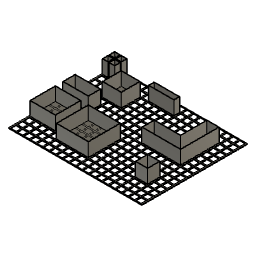
Grid (Autodesk Fusion 360 design; units mm, degrees)
Autodesk Fusion 360 part; units mm, degrees
note: some values were not read from the file. Set by a fixed rule: which face or edge a step refers to.
(part 1 of 2)
sketch "Sketch4" plane through (0, 0, 0) normal (0, 0, 1) x (1, 0, 0)
  line L0 (0, 0) -> (486, 0)
  line L1 (486, 0) -> (486, 385)
  line L2 (486, 385) -> (0, 385)
  line L3 (0, 385) -> (0, 0)
  line L4 (5, 2.5) -> (0, 2.5) construction
  line L5 (5, 2.5) -> (5, 0) construction
  line L6 (5, 2.5) -> (25, 2.5)
  line L7 (25, 2.5) -> (25, 22.5)
  line L8 (25, 22.5) -> (5, 22.5)
  line L9 (5, 22.5) -> (5, 2.5)
  line L10 (49, 22.5) -> (29, 22.5)
  line L11 (29, 22.5) -> (29, 2.5)
  line L12 (29, 2.5) -> (49, 2.5)
  line L13 (49, 2.5) -> (49, 22.5)
  line L14 (73, 22.5) -> (53, 22.5)
  line L15 (53, 22.5) -> (53, 2.5)
  line L16 (53, 2.5) -> (73, 2.5)
  line L17 (73, 2.5) -> (73, 22.5)
  line L18 (97, 22.5) -> (77, 22.5)
  line L19 (77, 22.5) -> (77, 2.5)
  line L20 (77, 2.5) -> (97, 2.5)
  line L21 (97, 2.5) -> (97, 22.5)
  line L22 (25, 46.5) -> (5, 46.5)
  line L23 (5, 46.5) -> (5, 26.5)
  line L24 (5, 26.5) -> (25, 26.5)
  line L25 (25, 26.5) -> (25, 46.5)
  line L26 (49, 46.5) -> (29, 46.5)
  line L27 (29, 46.5) -> (29, 26.5)
  line L28 (29, 26.5) -> (49, 26.5)
  line L29 (49, 26.5) -> (49, 46.5)
  line L30 (73, 46.5) -> (53, 46.5)
  line L31 (53, 46.5) -> (53, 26.5)
  line L32 (53, 26.5) -> (73, 26.5)
  line L33 (73, 26.5) -> (73, 46.5)
  line L34 (97, 46.5) -> (77, 46.5)
  line L35 (77, 46.5) -> (77, 26.5)
  line L36 (77, 26.5) -> (97, 26.5)
  line L37 (97, 26.5) -> (97, 46.5)
  line L38 (25, 70.5) -> (5, 70.5)
  line L39 (5, 70.5) -> (5, 50.5)
  line L40 (5, 50.5) -> (25, 50.5)
  line L41 (25, 50.5) -> (25, 70.5)
  line L42 (49, 70.5) -> (29, 70.5)
  line L43 (29, 70.5) -> (29, 50.5)
  line L44 (29, 50.5) -> (49, 50.5)
  line L45 (49, 50.5) -> (49, 70.5)
  line L46 (73, 70.5) -> (53, 70.5)
  line L47 (53, 70.5) -> (53, 50.5)
  line L48 (53, 50.5) -> (73, 50.5)
  line L49 (73, 50.5) -> (73, 70.5)
  line L50 (97, 70.5) -> (77, 70.5)
  line L51 (77, 70.5) -> (77, 50.5)
  line L52 (77, 50.5) -> (97, 50.5)
  line L53 (97, 50.5) -> (97, 70.5)
  line L54 (25, 94.5) -> (5, 94.5)
  line L55 (5, 94.5) -> (5, 74.5)
  line L56 (5, 74.5) -> (25, 74.5)
  line L57 (25, 74.5) -> (25, 94.5)
  line L58 (49, 94.5) -> (29, 94.5)
  line L59 (29, 94.5) -> (29, 74.5)
  line L60 (29, 74.5) -> (49, 74.5)
  line L61 (49, 74.5) -> (49, 94.5)
  line L62 (73, 94.5) -> (53, 94.5)
  line L63 (53, 94.5) -> (53, 74.5)
  line L64 (53, 74.5) -> (73, 74.5)
  line L65 (73, 74.5) -> (73, 94.5)
  line L66 (97, 94.5) -> (77, 94.5)
  line L67 (77, 94.5) -> (77, 74.5)
  line L68 (77, 74.5) -> (97, 74.5)
  line L69 (97, 74.5) -> (97, 94.5)
  line L70 (121, 22.5) -> (101, 22.5)
  line L71 (101, 22.5) -> (101, 2.5)
  line L72 (101, 2.5) -> (121, 2.5)
  line L73 (121, 2.5) -> (121, 22.5)
  line L74 (145, 22.5) -> (125, 22.5)
  line L75 (125, 22.5) -> (125, 2.5)
  line L76 (125, 2.5) -> (145, 2.5)
  line L77 (145, 2.5) -> (145, 22.5)
  line L78 (169, 22.5) -> (149, 22.5)
  line L79 (149, 22.5) -> (149, 2.5)
  line L80 (149, 2.5) -> (169, 2.5)
  line L81 (169, 2.5) -> (169, 22.5)
  line L82 (193, 22.5) -> (173, 22.5)
  line L83 (173, 22.5) -> (173, 2.5)
  line L84 (173, 2.5) -> (193, 2.5)
  line L85 (193, 2.5) -> (193, 22.5)
  line L86 (217, 22.5) -> (197, 22.5)
  line L87 (197, 22.5) -> (197, 2.5)
  line L88 (197, 2.5) -> (217, 2.5)
  line L89 (217, 2.5) -> (217, 22.5)
  line L90 (241, 22.5) -> (221, 22.5)
  line L91 (221, 22.5) -> (221, 2.5)
  line L92 (221, 2.5) -> (241, 2.5)
  line L93 (241, 2.5) -> (241, 22.5)
  line L94 (265, 22.5) -> (245, 22.5)
  line L95 (245, 22.5) -> (245, 2.5)
  line L96 (245, 2.5) -> (265, 2.5)
  line L97 (265, 2.5) -> (265, 22.5)
  line L98 (289, 22.5) -> (269, 22.5)
  line L99 (269, 22.5) -> (269, 2.5)
  line L100 (269, 2.5) -> (289, 2.5)
  line L101 (289, 2.5) -> (289, 22.5)
  line L102 (121, 46.5) -> (101, 46.5)
  line L103 (101, 46.5) -> (101, 26.5)
  line L104 (101, 26.5) -> (121, 26.5)
  line L105 (121, 26.5) -> (121, 46.5)
  line L106 (145, 46.5) -> (125, 46.5)
  line L107 (125, 46.5) -> (125, 26.5)
  line L108 (125, 26.5) -> (145, 26.5)
  line L109 (145, 26.5) -> (145, 46.5)
  line L110 (169, 46.5) -> (149, 46.5)
  line L111 (149, 46.5) -> (149, 26.5)
  line L112 (149, 26.5) -> (169, 26.5)
  line L113 (169, 26.5) -> (169, 46.5)
  line L114 (193, 46.5) -> (173, 46.5)
  line L115 (173, 46.5) -> (173, 26.5)
  line L116 (173, 26.5) -> (193, 26.5)
  line L117 (193, 26.5) -> (193, 46.5)
  line L118 (217, 46.5) -> (197, 46.5)
  line L119 (197, 46.5) -> (197, 26.5)
  line L120 (197, 26.5) -> (217, 26.5)
  line L121 (217, 26.5) -> (217, 46.5)
  line L122 (241, 46.5) -> (221, 46.5)
  line L123 (221, 46.5) -> (221, 26.5)
  line L124 (221, 26.5) -> (241, 26.5)
  line L125 (241, 26.5) -> (241, 46.5)
  line L126 (265, 46.5) -> (245, 46.5)
  line L127 (245, 46.5) -> (245, 26.5)
  line L128 (245, 26.5) -> (265, 26.5)
  line L129 (265, 26.5) -> (265, 46.5)
  line L130 (289, 46.5) -> (269, 46.5)
  line L131 (269, 46.5) -> (269, 26.5)
  line L132 (269, 26.5) -> (289, 26.5)
  line L133 (289, 26.5) -> (289, 46.5)
  line L134 (121, 70.5) -> (101, 70.5)
  line L135 (101, 70.5) -> (101, 50.5)
  line L136 (101, 50.5) -> (121, 50.5)
  line L137 (121, 50.5) -> (121, 70.5)
  line L138 (145, 70.5) -> (125, 70.5)
  line L139 (125, 70.5) -> (125, 50.5)
  line L140 (125, 50.5) -> (145, 50.5)
  line L141 (145, 50.5) -> (145, 70.5)
  line L142 (169, 70.5) -> (149, 70.5)
  line L143 (149, 70.5) -> (149, 50.5)
  line L144 (149, 50.5) -> (169, 50.5)
  line L145 (169, 50.5) -> (169, 70.5)
  line L146 (193, 70.5) -> (173, 70.5)
  line L147 (173, 70.5) -> (173, 50.5)
  line L148 (173, 50.5) -> (193, 50.5)
  line L149 (193, 50.5) -> (193, 70.5)
  line L150 (217, 70.5) -> (197, 70.5)
  line L151 (197, 70.5) -> (197, 50.5)
  line L152 (197, 50.5) -> (217, 50.5)
  line L153 (217, 50.5) -> (217, 70.5)
  line L154 (241, 70.5) -> (221, 70.5)
  line L155 (221, 70.5) -> (221, 50.5)
  line L156 (221, 50.5) -> (241, 50.5)
  line L157 (241, 50.5) -> (241, 70.5)
  line L158 (265, 70.5) -> (245, 70.5)
  line L159 (245, 70.5) -> (245, 50.5)
  line L160 (245, 50.5) -> (265, 50.5)
  line L161 (265, 50.5) -> (265, 70.5)
  line L162 (289, 70.5) -> (269, 70.5)
  line L163 (269, 70.5) -> (269, 50.5)
  line L164 (269, 50.5) -> (289, 50.5)
  line L165 (289, 50.5) -> (289, 70.5)
  line L166 (121, 94.5) -> (101, 94.5)
  line L167 (101, 94.5) -> (101, 74.5)
  line L168 (101, 74.5) -> (121, 74.5)
  line L169 (121, 74.5) -> (121, 94.5)
  line L170 (145, 94.5) -> (125, 94.5)
  line L171 (125, 94.5) -> (125, 74.5)
  line L172 (125, 74.5) -> (145, 74.5)
  line L173 (145, 74.5) -> (145, 94.5)
  line L174 (169, 94.5) -> (149, 94.5)
  line L175 (149, 94.5) -> (149, 74.5)
  line L176 (149, 74.5) -> (169, 74.5)
  line L177 (169, 74.5) -> (169, 94.5)
  line L178 (193, 94.5) -> (173, 94.5)
  line L179 (173, 94.5) -> (173, 74.5)
  line L180 (173, 74.5) -> (193, 74.5)
  line L181 (193, 74.5) -> (193, 94.5)
  line L182 (217, 94.5) -> (197, 94.5)
  line L183 (197, 94.5) -> (197, 74.5)
  line L184 (197, 74.5) -> (217, 74.5)
  line L185 (217, 74.5) -> (217, 94.5)
  line L186 (241, 94.5) -> (221, 94.5)
  line L187 (221, 94.5) -> (221, 74.5)
  line L188 (221, 74.5) -> (241, 74.5)
  line L189 (241, 74.5) -> (241, 94.5)
  line L190 (265, 94.5) -> (245, 94.5)
  line L191 (245, 94.5) -> (245, 74.5)
  line L192 (245, 74.5) -> (265, 74.5)
  line L193 (265, 74.5) -> (265, 94.5)
  line L194 (289, 94.5) -> (269, 94.5)
  line L195 (269, 94.5) -> (269, 74.5)
  line L196 (269, 74.5) -> (289, 74.5)
  line L197 (289, 74.5) -> (289, 94.5)
  line L198 (25, 118.5) -> (5, 118.5)
  line L199 (5, 118.5) -> (5, 98.5)
  line L200 (5, 98.5) -> (25, 98.5)
  line L201 (25, 98.5) -> (25, 118.5)
  line L202 (49, 118.5) -> (29, 118.5)
  line L203 (29, 118.5) -> (29, 98.5)
  line L204 (29, 98.5) -> (49, 98.5)
  line L205 (49, 98.5) -> (49, 118.5)
  line L206 (73, 118.5) -> (53, 118.5)
  line L207 (53, 118.5) -> (53, 98.5)
  line L208 (53, 98.5) -> (73, 98.5)
  line L209 (73, 98.5) -> (73, 118.5)
  line L210 (97, 118.5) -> (77, 118.5)
  line L211 (77, 118.5) -> (77, 98.5)
  line L212 (77, 98.5) -> (97, 98.5)
  line L213 (97, 98.5) -> (97, 118.5)
  line L214 (121, 118.5) -> (101, 118.5)
  line L215 (101, 118.5) -> (101, 98.5)
  line L216 (101, 98.5) -> (121, 98.5)
  line L217 (121, 98.5) -> (121, 118.5)
  line L218 (145, 118.5) -> (125, 118.5)
  line L219 (125, 118.5) -> (125, 98.5)
  line L220 (125, 98.5) -> (145, 98.5)
  line L221 (145, 98.5) -> (145, 118.5)
  line L222 (169, 118.5) -> (149, 118.5)
  line L223 (149, 118.5) -> (149, 98.5)
  line L224 (149, 98.5) -> (169, 98.5)
  line L225 (169, 98.5) -> (169, 118.5)
  line L226 (193, 118.5) -> (173, 118.5)
  line L227 (173, 118.5) -> (173, 98.5)
  line L228 (173, 98.5) -> (193, 98.5)
  line L229 (193, 98.5) -> (193, 118.5)
  line L230 (217, 118.5) -> (197, 118.5)
  line L231 (197, 118.5) -> (197, 98.5)
  line L232 (197, 98.5) -> (217, 98.5)
  line L233 (217, 98.5) -> (217, 118.5)
  line L234 (241, 118.5) -> (221, 118.5)
  line L235 (221, 118.5) -> (221, 98.5)
  line L236 (221, 98.5) -> (241, 98.5)
  line L237 (241, 98.5) -> (241, 118.5)
  line L238 (265, 118.5) -> (245, 118.5)
  line L239 (245, 118.5) -> (245, 98.5)
  line L240 (245, 98.5) -> (265, 98.5)
  line L241 (265, 98.5) -> (265, 118.5)
  line L242 (289, 118.5) -> (269, 118.5)
  line L243 (269, 118.5) -> (269, 98.5)
  line L244 (269, 98.5) -> (289, 98.5)
  line L245 (289, 98.5) -> (289, 118.5)
  line L246 (25, 142.5) -> (5, 142.5)
  line L247 (5, 142.5) -> (5, 122.5)
  line L248 (5, 122.5) -> (25, 122.5)
  line L249 (25, 122.5) -> (25, 142.5)
  line L250 (49, 142.5) -> (29, 142.5)
  line L251 (29, 142.5) -> (29, 122.5)
  line L252 (29, 122.5) -> (49, 122.5)
  line L253 (49, 122.5) -> (49, 142.5)
  line L254 (73, 142.5) -> (53, 142.5)
  line L255 (53, 142.5) -> (53, 122.5)
  line L256 (53, 122.5) -> (73, 122.5)
  line L257 (73, 122.5) -> (73, 142.5)
  line L258 (97, 142.5) -> (77, 142.5)
  line L259 (77, 142.5) -> (77, 122.5)
  line L260 (77, 122.5) -> (97, 122.5)
  line L261 (97, 122.5) -> (97, 142.5)
  line L262 (121, 142.5) -> (101, 142.5)
  line L263 (101, 142.5) -> (101, 122.5)
  line L264 (101, 122.5) -> (121, 122.5)
  line L265 (121, 122.5) -> (121, 142.5)
  line L266 (145, 142.5) -> (125, 142.5)
  line L267 (125, 142.5) -> (125, 122.5)
  line L268 (125, 122.5) -> (145, 122.5)
  line L269 (145, 122.5) -> (145, 142.5)
  line L270 (169, 142.5) -> (149, 142.5)
  line L271 (149, 142.5) -> (149, 122.5)
  line L272 (149, 122.5) -> (169, 122.5)
  line L273 (169, 122.5) -> (169, 142.5)
  line L274 (193, 142.5) -> (173, 142.5)
  line L275 (173, 142.5) -> (173, 122.5)
  line L276 (173, 122.5) -> (193, 122.5)
  line L277 (193, 122.5) -> (193, 142.5)
  line L278 (217, 142.5) -> (197, 142.5)
  line L279 (197, 142.5) -> (197, 122.5)
  line L280 (197, 122.5) -> (217, 122.5)
  line L281 (217, 122.5) -> (217, 142.5)
  line L282 (241, 142.5) -> (221, 142.5)
  line L283 (221, 142.5) -> (221, 122.5)
  line L284 (221, 122.5) -> (241, 122.5)
  line L285 (241, 122.5) -> (241, 142.5)
  line L286 (265, 142.5) -> (245, 142.5)
  line L287 (245, 142.5) -> (245, 122.5)
  line L288 (245, 122.5) -> (265, 122.5)
  line L289 (265, 122.5) -> (265, 142.5)
  line L290 (289, 142.5) -> (269, 142.5)
  line L291 (269, 142.5) -> (269, 122.5)
  line L292 (269, 122.5) -> (289, 122.5)
  line L293 (289, 122.5) -> (289, 142.5)
  line L294 (25, 166.5) -> (5, 166.5)
  line L295 (5, 166.5) -> (5, 146.5)
  line L296 (5, 146.5) -> (25, 146.5)
  line L297 (25, 146.5) -> (25, 166.5)
  line L298 (49, 166.5) -> (29, 166.5)
  line L299 (29, 166.5) -> (29, 146.5)
  line L300 (29, 146.5) -> (49, 146.5)
  line L301 (49, 146.5) -> (49, 166.5)
  line L302 (73, 166.5) -> (53, 166.5)
  line L303 (53, 166.5) -> (53, 146.5)
  line L304 (53, 146.5) -> (73, 146.5)
  line L305 (73, 146.5) -> (73, 166.5)
  line L306 (97, 166.5) -> (77, 166.5)
  line L307 (77, 166.5) -> (77, 146.5)
  line L308 (77, 146.5) -> (97, 146.5)
  line L309 (97, 146.5) -> (97, 166.5)
  line L310 (121, 166.5) -> (101, 166.5)
  line L311 (101, 166.5) -> (101, 146.5)
  line L312 (101, 146.5) -> (121, 146.5)
  line L313 (121, 146.5) -> (121, 166.5)
  line L314 (145, 166.5) -> (125, 166.5)
  line L315 (125, 166.5) -> (125, 146.5)
  line L316 (125, 146.5) -> (145, 146.5)
  line L317 (145, 146.5) -> (145, 166.5)
  line L318 (169, 166.5) -> (149, 166.5)
  line L319 (149, 166.5) -> (149, 146.5)
  line L320 (149, 146.5) -> (169, 146.5)
  line L321 (169, 146.5) -> (169, 166.5)
  line L322 (193, 166.5) -> (173, 166.5)
  line L323 (173, 166.5) -> (173, 146.5)
  line L324 (173, 146.5) -> (193, 146.5)
  line L325 (193, 146.5) -> (193, 166.5)
  line L326 (217, 166.5) -> (197, 166.5)
  line L327 (197, 166.5) -> (197, 146.5)
  line L328 (197, 146.5) -> (217, 146.5)
  line L329 (217, 146.5) -> (217, 166.5)
  line L330 (241, 166.5) -> (221, 166.5)
  line L331 (221, 166.5) -> (221, 146.5)
  line L332 (221, 146.5) -> (241, 146.5)
  line L333 (241, 146.5) -> (241, 166.5)
  line L334 (265, 166.5) -> (245, 166.5)
  line L335 (245, 166.5) -> (245, 146.5)
  line L336 (245, 146.5) -> (265, 146.5)
  line L337 (265, 146.5) -> (265, 166.5)
  line L338 (289, 166.5) -> (269, 166.5)
  line L339 (269, 166.5) -> (269, 146.5)
  line L340 (269, 146.5) -> (289, 146.5)
  line L341 (289, 146.5) -> (289, 166.5)
  line L342 (25, 190.5) -> (5, 190.5)
  line L343 (5, 190.5) -> (5, 170.5)
  line L344 (5, 170.5) -> (25, 170.5)
  line L345 (25, 170.5) -> (25, 190.5)
  line L346 (49, 190.5) -> (29, 190.5)
  line L347 (29, 190.5) -> (29, 170.5)
  line L348 (29, 170.5) -> (49, 170.5)
  line L349 (49, 170.5) -> (49, 190.5)
  line L350 (73, 190.5) -> (53, 190.5)
  line L351 (53, 190.5) -> (53, 170.5)
  line L352 (53, 170.5) -> (73, 170.5)
  line L353 (73, 170.5) -> (73, 190.5)
  line L354 (97, 190.5) -> (77, 190.5)
  line L355 (77, 190.5) -> (77, 170.5)
  line L356 (77, 170.5) -> (97, 170.5)
  line L357 (97, 170.5) -> (97, 190.5)
  line L358 (121, 190.5) -> (101, 190.5)
  line L359 (101, 190.5) -> (101, 170.5)
  line L360 (101, 170.5) -> (121, 170.5)
  line L361 (121, 170.5) -> (121, 190.5)
  line L362 (145, 190.5) -> (125, 190.5)
  line L363 (125, 190.5) -> (125, 170.5)
  line L364 (125, 170.5) -> (145, 170.5)
  line L365 (145, 170.5) -> (145, 190.5)
  line L366 (169, 190.5) -> (149, 190.5)
  line L367 (149, 190.5) -> (149, 170.5)
  line L368 (149, 170.5) -> (169, 170.5)
  line L369 (169, 170.5) -> (169, 190.5)
  line L370 (193, 190.5) -> (173, 190.5)
  line L371 (173, 190.5) -> (173, 170.5)
  line L372 (173, 170.5) -> (193, 170.5)
  line L373 (193, 170.5) -> (193, 190.5)
  line L374 (217, 190.5) -> (197, 190.5)
  line L375 (197, 190.5) -> (197, 170.5)
  line L376 (197, 170.5) -> (217, 170.5)
  line L377 (217, 170.5) -> (217, 190.5)
  line L378 (241, 190.5) -> (221, 190.5)
  line L379 (221, 190.5) -> (221, 170.5)
  line L380 (221, 170.5) -> (241, 170.5)
  line L381 (241, 170.5) -> (241, 190.5)
  line L382 (265, 190.5) -> (245, 190.5)
  line L383 (245, 190.5) -> (245, 170.5)
  line L384 (245, 170.5) -> (265, 170.5)
  line L385 (265, 170.5) -> (265, 190.5)
  line L386 (289, 190.5) -> (269, 190.5)
  line L387 (269, 190.5) -> (269, 170.5)
  line L388 (269, 170.5) -> (289, 170.5)
  line L389 (289, 170.5) -> (289, 190.5)
  line L390 (25, 214.5) -> (5, 214.5)
  line L391 (5, 214.5) -> (5, 194.5)
  line L392 (5, 194.5) -> (25, 194.5)
  line L393 (25, 194.5) -> (25, 214.5)
  line L394 (49, 214.5) -> (29, 214.5)
  line L395 (29, 214.5) -> (29, 194.5)
  line L396 (29, 194.5) -> (49, 194.5)
  line L397 (49, 194.5) -> (49, 214.5)
  line L398 (73, 214.5) -> (53, 214.5)
  line L399 (53, 214.5) -> (53, 194.5)
  line L400 (53, 194.5) -> (73, 194.5)
  line L401 (73, 194.5) -> (73, 214.5)
  line L402 (97, 214.5) -> (77, 214.5)
  line L403 (77, 214.5) -> (77, 194.5)
  line L404 (77, 194.5) -> (97, 194.5)
  line L405 (97, 194.5) -> (97, 214.5)
  line L406 (121, 214.5) -> (101, 214.5)
  line L407 (101, 214.5) -> (101, 194.5)
  line L408 (101, 194.5) -> (121, 194.5)
  line L409 (121, 194.5) -> (121, 214.5)
  line L410 (145, 214.5) -> (125, 214.5)
  line L411 (125, 214.5) -> (125, 194.5)
  line L412 (125, 194.5) -> (145, 194.5)
  line L413 (145, 194.5) -> (145, 214.5)
  line L414 (169, 214.5) -> (149, 214.5)
  line L415 (149, 214.5) -> (149, 194.5)
  line L416 (149, 194.5) -> (169, 194.5)
  line L417 (169, 194.5) -> (169, 214.5)
  line L418 (193, 214.5) -> (173, 214.5)
  line L419 (173, 214.5) -> (173, 194.5)
  line L420 (173, 194.5) -> (193, 194.5)
  line L421 (193, 194.5) -> (193, 214.5)
  line L422 (217, 214.5) -> (197, 214.5)
  line L423 (197, 214.5) -> (197, 194.5)
  line L424 (197, 194.5) -> (217, 194.5)
  line L425 (217, 194.5) -> (217, 214.5)
  line L426 (241, 214.5) -> (221, 214.5)
  line L427 (221, 214.5) -> (221, 194.5)
  line L428 (221, 194.5) -> (241, 194.5)
  line L429 (241, 194.5) -> (241, 214.5)
  line L430 (265, 214.5) -> (245, 214.5)
  line L431 (245, 214.5) -> (245, 194.5)
  line L432 (245, 194.5) -> (265, 194.5)
  line L433 (265, 194.5) -> (265, 214.5)
  line L434 (289, 214.5) -> (269, 214.5)
  line L435 (269, 214.5) -> (269, 194.5)
  line L436 (269, 194.5) -> (289, 194.5)
  line L437 (289, 194.5) -> (289, 214.5)
  line L438 (25, 238.5) -> (5, 238.5)
  line L439 (5, 238.5) -> (5, 218.5)
  line L440 (5, 218.5) -> (25, 218.5)
  line L441 (25, 218.5) -> (25, 238.5)
  line L442 (49, 238.5) -> (29, 238.5)
  line L443 (29, 238.5) -> (29, 218.5)
  line L444 (29, 218.5) -> (49, 218.5)
  line L445 (49, 218.5) -> (49, 238.5)
  line L446 (73, 238.5) -> (53, 238.5)
  line L447 (53, 238.5) -> (53, 218.5)
  line L448 (53, 218.5) -> (73, 218.5)
  line L449 (73, 218.5) -> (73, 238.5)
  line L450 (97, 238.5) -> (77, 238.5)
  line L451 (77, 238.5) -> (77, 218.5)
  line L452 (77, 218.5) -> (97, 218.5)
  line L453 (97, 218.5) -> (97, 238.5)
  line L454 (121, 238.5) -> (101, 238.5)
  line L455 (101, 238.5) -> (101, 218.5)
  line L456 (101, 218.5) -> (121, 218.5)
  line L457 (121, 218.5) -> (121, 238.5)
  line L458 (145, 238.5) -> (125, 238.5)
  line L459 (125, 238.5) -> (125, 218.5)
  line L460 (125, 218.5) -> (145, 218.5)
  line L461 (145, 218.5) -> (145, 238.5)
  line L462 (169, 238.5) -> (149, 238.5)
  line L463 (149, 238.5) -> (149, 218.5)
  line L464 (149, 218.5) -> (169, 218.5)
  line L465 (169, 218.5) -> (169, 238.5)
  line L466 (193, 238.5) -> (173, 238.5)
  line L467 (173, 238.5) -> (173, 218.5)
  line L468 (173, 218.5) -> (193, 218.5)
  line L469 (193, 218.5) -> (193, 238.5)
  line L470 (217, 238.5) -> (197, 238.5)
  line L471 (197, 238.5) -> (197, 218.5)
  line L472 (197, 218.5) -> (217, 218.5)
  line L473 (217, 218.5) -> (217, 238.5)
  line L474 (241, 238.5) -> (221, 238.5)
  line L475 (221, 238.5) -> (221, 218.5)
  line L476 (221, 218.5) -> (241, 218.5)
  line L477 (241, 218.5) -> (241, 238.5)
  line L478 (265, 238.5) -> (245, 238.5)
  line L479 (245, 238.5) -> (245, 218.5)
  line L480 (245, 218.5) -> (265, 218.5)
  line L481 (265, 218.5) -> (265, 238.5)
  line L482 (289, 238.5) -> (269, 238.5)
  line L483 (269, 238.5) -> (269, 218.5)
  line L484 (269, 218.5) -> (289, 218.5)
  line L485 (289, 218.5) -> (289, 238.5)
  line L486 (25, 262.5) -> (5, 262.5)
  line L487 (5, 262.5) -> (5, 242.5)
  line L488 (5, 242.5) -> (25, 242.5)
  line L489 (25, 242.5) -> (25, 262.5)
  line L490 (49, 262.5) -> (29, 262.5)
  line L491 (29, 262.5) -> (29, 242.5)
  line L492 (29, 242.5) -> (49, 242.5)
  line L493 (49, 242.5) -> (49, 262.5)
  line L494 (73, 262.5) -> (53, 262.5)
  line L495 (53, 262.5) -> (53, 242.5)
  line L496 (53, 242.5) -> (73, 242.5)
  line L497 (73, 242.5) -> (73, 262.5)
  line L498 (97, 262.5) -> (77, 262.5)
  line L499 (77, 262.5) -> (77, 242.5)
  line L500 (77, 242.5) -> (97, 242.5)
  line L501 (97, 242.5) -> (97, 262.5)
  line L502 (121, 262.5) -> (101, 262.5)
  line L503 (101, 262.5) -> (101, 242.5)
  line L504 (101, 242.5) -> (121, 242.5)
  line L505 (121, 242.5) -> (121, 262.5)
  line L506 (145, 262.5) -> (125, 262.5)
  line L507 (125, 262.5) -> (125, 242.5)
  line L508 (125, 242.5) -> (145, 242.5)
  line L509 (145, 242.5) -> (145, 262.5)
  line L510 (169, 262.5) -> (149, 262.5)
  line L511 (149, 262.5) -> (149, 242.5)
  line L512 (149, 242.5) -> (169, 242.5)
  line L513 (169, 242.5) -> (169, 262.5)
  line L514 (193, 262.5) -> (173, 262.5)
  line L515 (173, 262.5) -> (173, 242.5)
  line L516 (173, 242.5) -> (193, 242.5)
  line L517 (193, 242.5) -> (193, 262.5)
  line L518 (217, 262.5) -> (197, 262.5)
  line L519 (197, 262.5) -> (197, 242.5)
  line L520 (197, 242.5) -> (217, 242.5)
  line L521 (217, 242.5) -> (217, 262.5)
  line L522 (241, 262.5) -> (221, 262.5)
  line L523 (221, 262.5) -> (221, 242.5)
  line L524 (221, 242.5) -> (241, 242.5)
  line L525 (241, 242.5) -> (241, 262.5)
  line L526 (265, 262.5) -> (245, 262.5)
  line L527 (245, 262.5) -> (245, 242.5)
  line L528 (245, 242.5) -> (265, 242.5)
  line L529 (265, 242.5) -> (265, 262.5)
  line L530 (289, 262.5) -> (269, 262.5)
  line L531 (269, 262.5) -> (269, 242.5)
  line L532 (269, 242.5) -> (289, 242.5)
  line L533 (289, 242.5) -> (289, 262.5)
  line L534 (25, 286.5) -> (5, 286.5)
  line L535 (5, 286.5) -> (5, 266.5)
  line L536 (5, 266.5) -> (25, 266.5)
  line L537 (25, 266.5) -> (25, 286.5)
  line L538 (49, 286.5) -> (29, 286.5)
  line L539 (29, 286.5) -> (29, 266.5)
  line L540 (29, 266.5) -> (49, 266.5)
  line L541 (49, 266.5) -> (49, 286.5)
  line L542 (73, 286.5) -> (53, 286.5)
  line L543 (53, 286.5) -> (53, 266.5)
  line L544 (53, 266.5) -> (73, 266.5)
  line L545 (73, 266.5) -> (73, 286.5)
  line L546 (97, 286.5) -> (77, 286.5)
  line L547 (77, 286.5) -> (77, 266.5)
  line L548 (77, 266.5) -> (97, 266.5)
  line L549 (97, 266.5) -> (97, 286.5)
  line L550 (121, 286.5) -> (101, 286.5)
  line L551 (101, 286.5) -> (101, 266.5)
  line L552 (101, 266.5) -> (121, 266.5)
  line L553 (121, 266.5) -> (121, 286.5)
  line L554 (145, 286.5) -> (125, 286.5)
  line L555 (125, 286.5) -> (125, 266.5)
  line L556 (125, 266.5) -> (145, 266.5)
  line L557 (145, 266.5) -> (145, 286.5)
  line L558 (169, 286.5) -> (149, 286.5)
  line L559 (149, 286.5) -> (149, 266.5)
  line L560 (149, 266.5) -> (169, 266.5)
  line L561 (169, 266.5) -> (169, 286.5)
  line L562 (193, 286.5) -> (173, 286.5)
  line L563 (173, 286.5) -> (173, 266.5)
  line L564 (173, 266.5) -> (193, 266.5)
  line L565 (193, 266.5) -> (193, 286.5)
  line L566 (217, 286.5) -> (197, 286.5)
  line L567 (197, 286.5) -> (197, 266.5)
  line L568 (197, 266.5) -> (217, 266.5)
  line L569 (217, 266.5) -> (217, 286.5)
  line L570 (241, 286.5) -> (221, 286.5)
  line L571 (221, 286.5) -> (221, 266.5)
  line L572 (221, 266.5) -> (241, 266.5)
  line L573 (241, 266.5) -> (241, 286.5)
  line L574 (265, 286.5) -> (245, 286.5)
  line L575 (245, 286.5) -> (245, 266.5)
  line L576 (245, 266.5) -> (265, 266.5)
  line L577 (265, 266.5) -> (265, 286.5)
  line L578 (289, 286.5) -> (269, 286.5)
  line L579 (269, 286.5) -> (269, 266.5)
  line L580 (269, 266.5) -> (289, 266.5)
  line L581 (289, 266.5) -> (289, 286.5)
  line L582 (25, 310.5) -> (5, 310.5)
  line L583 (5, 310.5) -> (5, 290.5)
  line L584 (5, 290.5) -> (25, 290.5)
  line L585 (25, 290.5) -> (25, 310.5)
  line L586 (49, 310.5) -> (29, 310.5)
  line L587 (29, 310.5) -> (29, 290.5)
  line L588 (29, 290.5) -> (49, 290.5)
  line L589 (49, 290.5) -> (49, 310.5)
  line L590 (73, 310.5) -> (53, 310.5)
  line L591 (53, 310.5) -> (53, 290.5)
  line L592 (53, 290.5) -> (73, 290.5)
  line L593 (73, 290.5) -> (73, 310.5)
  line L594 (97, 310.5) -> (77, 310.5)
  line L595 (77, 310.5) -> (77, 290.5)
  line L596 (77, 290.5) -> (97, 290.5)
  line L597 (97, 290.5) -> (97, 310.5)
  line L598 (121, 310.5) -> (101, 310.5)
  line L599 (101, 310.5) -> (101, 290.5)
  line L600 (101, 290.5) -> (121, 290.5)
  line L601 (121, 290.5) -> (121, 310.5)
  line L602 (145, 310.5) -> (125, 310.5)
  line L603 (125, 310.5) -> (125, 290.5)
  line L604 (125, 290.5) -> (145, 290.5)
  line L605 (145, 290.5) -> (145, 310.5)
  line L606 (169, 310.5) -> (149, 310.5)
  line L607 (149, 310.5) -> (149, 290.5)
  line L608 (149, 290.5) -> (169, 290.5)
  line L609 (169, 290.5) -> (169, 310.5)
  line L610 (193, 310.5) -> (173, 310.5)
  line L611 (173, 310.5) -> (173, 290.5)
  line L612 (173, 290.5) -> (193, 290.5)
  line L613 (193, 290.5) -> (193, 310.5)
  line L614 (217, 310.5) -> (197, 310.5)
  line L615 (197, 310.5) -> (197, 290.5)
  line L616 (197, 290.5) -> (217, 290.5)
  line L617 (217, 290.5) -> (217, 310.5)
  line L618 (241, 310.5) -> (221, 310.5)
  line L619 (221, 310.5) -> (221, 290.5)
  line L620 (221, 290.5) -> (241, 290.5)
  line L621 (241, 290.5) -> (241, 310.5)
  line L622 (265, 310.5) -> (245, 310.5)
  line L623 (245, 310.5) -> (245, 290.5)
  line L624 (245, 290.5) -> (265, 290.5)
  line L625 (265, 290.5) -> (265, 310.5)
  line L626 (289, 310.5) -> (269, 310.5)
  line L627 (269, 310.5) -> (269, 290.5)
  line L628 (269, 290.5) -> (289, 290.5)
  line L629 (289, 290.5) -> (289, 310.5)
  line L630 (25, 334.5) -> (5, 334.5)
  line L631 (5, 334.5) -> (5, 314.5)
  line L632 (5, 314.5) -> (25, 314.5)
  line L633 (25, 314.5) -> (25, 334.5)
  line L634 (49, 334.5) -> (29, 334.5)
  line L635 (29, 334.5) -> (29, 314.5)
  line L636 (29, 314.5) -> (49, 314.5)
  line L637 (49, 314.5) -> (49, 334.5)
  line L638 (73, 334.5) -> (53, 334.5)
  line L639 (53, 334.5) -> (53, 314.5)
  line L640 (53, 314.5) -> (73, 314.5)
  line L641 (73, 314.5) -> (73, 334.5)
  line L642 (97, 334.5) -> (77, 334.5)
  line L643 (77, 334.5) -> (77, 314.5)
  line L644 (77, 314.5) -> (97, 314.5)
  line L645 (97, 314.5) -> (97, 334.5)
  line L646 (121, 334.5) -> (101, 334.5)
  line L647 (101, 334.5) -> (101, 314.5)
  line L648 (101, 314.5) -> (121, 314.5)
  line L649 (121, 314.5) -> (121, 334.5)
  line L650 (145, 334.5) -> (125, 334.5)
  line L651 (125, 334.5) -> (125, 314.5)
  line L652 (125, 314.5) -> (145, 314.5)
  line L653 (145, 314.5) -> (145, 334.5)
  line L654 (169, 334.5) -> (149, 334.5)
  line L655 (149, 334.5) -> (149, 314.5)
  line L656 (149, 314.5) -> (169, 314.5)
  line L657 (169, 314.5) -> (169, 334.5)
  line L658 (193, 334.5) -> (173, 334.5)
  line L659 (173, 334.5) -> (173, 314.5)
  line L660 (173, 314.5) -> (193, 314.5)
  line L661 (193, 314.5) -> (193, 334.5)
  line L662 (217, 334.5) -> (197, 334.5)
  line L663 (197, 334.5) -> (197, 314.5)
  line L664 (197, 314.5) -> (217, 314.5)
  line L665 (217, 314.5) -> (217, 334.5)
  line L666 (241, 334.5) -> (221, 334.5)
  line L667 (221, 334.5) -> (221, 314.5)
  line L668 (221, 314.5) -> (241, 314.5)
  line L669 (241, 314.5) -> (241, 334.5)
  line L670 (265, 334.5) -> (245, 334.5)
  line L671 (245, 334.5) -> (245, 314.5)
  line L672 (245, 314.5) -> (265, 314.5)
  line L673 (265, 314.5) -> (265, 334.5)
  line L674 (289, 334.5) -> (269, 334.5)
  line L675 (269, 334.5) -> (269, 314.5)
  line L676 (269, 314.5) -> (289, 314.5)
  line L677 (289, 314.5) -> (289, 334.5)
  line L678 (25, 358.5) -> (5, 358.5)
  line L679 (5, 358.5) -> (5, 338.5)
  line L680 (5, 338.5) -> (25, 338.5)
  line L681 (25, 338.5) -> (25, 358.5)
  line L682 (49, 358.5) -> (29, 358.5)
  line L683 (29, 358.5) -> (29, 338.5)
  line L684 (29, 338.5) -> (49, 338.5)
  line L685 (49, 338.5) -> (49, 358.5)
  line L686 (73, 358.5) -> (53, 358.5)
  line L687 (53, 358.5) -> (53, 338.5)
  line L688 (53, 338.5) -> (73, 338.5)
  line L689 (73, 338.5) -> (73, 358.5)
  line L690 (97, 358.5) -> (77, 358.5)
  line L691 (77, 358.5) -> (77, 338.5)
  line L692 (77, 338.5) -> (97, 338.5)
  line L693 (97, 338.5) -> (97, 358.5)
  line L694 (121, 358.5) -> (101, 358.5)
  line L695 (101, 358.5) -> (101, 338.5)
  line L696 (101, 338.5) -> (121, 338.5)
  line L697 (121, 338.5) -> (121, 358.5)
  line L698 (145, 358.5) -> (125, 358.5)
  line L699 (125, 358.5) -> (125, 338.5)
  line L700 (125, 338.5) -> (145, 338.5)
  line L701 (145, 338.5) -> (145, 358.5)
  line L702 (169, 358.5) -> (149, 358.5)
  line L703 (149, 358.5) -> (149, 338.5)
  line L704 (149, 338.5) -> (169, 338.5)
  line L705 (169, 338.5) -> (169, 358.5)
  line L706 (193, 358.5) -> (173, 358.5)
  line L707 (173, 358.5) -> (173, 338.5)
  line L708 (173, 338.5) -> (193, 338.5)
  line L709 (193, 338.5) -> (193, 358.5)
  line L710 (217, 358.5) -> (197, 358.5)
  line L711 (197, 358.5) -> (197, 338.5)
  line L712 (197, 338.5) -> (217, 338.5)
  line L713 (217, 338.5) -> (217, 358.5)
  line L714 (241, 358.5) -> (221, 358.5)
  line L715 (221, 358.5) -> (221, 338.5)
  line L716 (221, 338.5) -> (241, 338.5)
  line L717 (241, 338.5) -> (241, 358.5)
  line L718 (265, 358.5) -> (245, 358.5)
  line L719 (245, 358.5) -> (245, 338.5)
  line L720 (245, 338.5) -> (265, 338.5)
  line L721 (265, 338.5) -> (265, 358.5)
  line L722 (289, 358.5) -> (269, 358.5)
  line L723 (269, 358.5) -> (269, 338.5)
  line L724 (269, 338.5) -> (289, 338.5)
  line L725 (289, 338.5) -> (289, 358.5)
  line L726 (25, 382.5) -> (5, 382.5)
  line L727 (5, 382.5) -> (5, 362.5)
  line L728 (5, 362.5) -> (25, 362.5)
  line L729 (25, 362.5) -> (25, 382.5)
  line L730 (49, 382.5) -> (29, 382.5)
  line L731 (29, 382.5) -> (29, 362.5)
  line L732 (29, 362.5) -> (49, 362.5)
  line L733 (49, 362.5) -> (49, 382.5)
  line L734 (73, 382.5) -> (53, 382.5)
  line L735 (53, 382.5) -> (53, 362.5)
  line L736 (53, 362.5) -> (73, 362.5)
  line L737 (73, 362.5) -> (73, 382.5)
  line L738 (97, 382.5) -> (77, 382.5)
  line L739 (77, 382.5) -> (77, 362.5)
  line L740 (77, 362.5) -> (97, 362.5)
  line L741 (97, 362.5) -> (97, 382.5)
  line L742 (121, 382.5) -> (101, 382.5)
  line L743 (101, 382.5) -> (101, 362.5)
  line L744 (101, 362.5) -> (121, 362.5)
  line L745 (121, 362.5) -> (121, 382.5)
  line L746 (145, 382.5) -> (125, 382.5)
  line L747 (125, 382.5) -> (125, 362.5)
  line L748 (125, 362.5) -> (145, 362.5)
  line L749 (145, 362.5) -> (145, 382.5)
  line L750 (169, 382.5) -> (149, 382.5)
  line L751 (149, 382.5) -> (149, 362.5)
  line L752 (149, 362.5) -> (169, 362.5)
  line L753 (169, 362.5) -> (169, 382.5)
  line L754 (193, 382.5) -> (173, 382.5)
  line L755 (173, 382.5) -> (173, 362.5)
  line L756 (173, 362.5) -> (193, 362.5)
  line L757 (193, 362.5) -> (193, 382.5)
  line L758 (217, 382.5) -> (197, 382.5)
  line L759 (197, 382.5) -> (197, 362.5)
  line L760 (197, 362.5) -> (217, 362.5)
  line L761 (217, 362.5) -> (217, 382.5)
  line L762 (241, 382.5) -> (221, 382.5)
  line L763 (221, 382.5) -> (221, 362.5)
  line L764 (221, 362.5) -> (241, 362.5)
  line L765 (241, 362.5) -> (241, 382.5)
  line L766 (265, 382.5) -> (245, 382.5)
  line L767 (245, 382.5) -> (245, 362.5)
  line L768 (245, 362.5) -> (265, 362.5)
  line L769 (265, 362.5) -> (265, 382.5)
  line L770 (289, 382.5) -> (269, 382.5)
  line L771 (269, 382.5) -> (269, 362.5)
  line L772 (269, 362.5) -> (289, 362.5)
  line L773 (289, 362.5) -> (289, 382.5)
  line L774 (313, 22.5) -> (293, 22.5)
  line L775 (293, 22.5) -> (293, 2.5)
  line L776 (293, 2.5) -> (313, 2.5)
  line L777 (313, 2.5) -> (313, 22.5)
  line L778 (337, 22.5) -> (317, 22.5)
  line L779 (317, 22.5) -> (317, 2.5)
  line L780 (317, 2.5) -> (337, 2.5)
  line L781 (337, 2.5) -> (337, 22.5)
  line L782 (361, 22.5) -> (341, 22.5)
  line L783 (341, 22.5) -> (341, 2.5)
  line L784 (341, 2.5) -> (361, 2.5)
  line L785 (361, 2.5) -> (361, 22.5)
  line L786 (385, 22.5) -> (365, 22.5)
  line L787 (365, 22.5) -> (365, 2.5)
  line L788 (365, 2.5) -> (385, 2.5)
  line L789 (385, 2.5) -> (385, 22.5)
  line L790 (409, 22.5) -> (389, 22.5)
  line L791 (389, 22.5) -> (389, 2.5)
  line L792 (389, 2.5) -> (409, 2.5)
  line L793 (409, 2.5) -> (409, 22.5)
  line L794 (433, 22.5) -> (413, 22.5)
  line L795 (413, 22.5) -> (413, 2.5)
  line L796 (413, 2.5) -> (433, 2.5)
  line L797 (433, 2.5) -> (433, 22.5)
  line L798 (457, 22.5) -> (437, 22.5)
  line L799 (437, 22.5) -> (437, 2.5)
  line L800 (437, 2.5) -> (457, 2.5)
  line L801 (457, 2.5) -> (457, 22.5)
  line L802 (481, 22.5) -> (461, 22.5)
  line L803 (461, 22.5) -> (461, 2.5)
  line L804 (461, 2.5) -> (481, 2.5)
  line L805 (481, 2.5) -> (481, 22.5)
  line L806 (313, 46.5) -> (293, 46.5)
  line L807 (293, 46.5) -> (293, 26.5)
  line L808 (293, 26.5) -> (313, 26.5)
  line L809 (313, 26.5) -> (313, 46.5)
  line L810 (337, 46.5) -> (317, 46.5)
  line L811 (317, 46.5) -> (317, 26.5)
  line L812 (317, 26.5) -> (337, 26.5)
  line L813 (337, 26.5) -> (337, 46.5)
  line L814 (361, 46.5) -> (341, 46.5)
  line L815 (341, 46.5) -> (341, 26.5)
  line L816 (341, 26.5) -> (361, 26.5)
  line L817 (361, 26.5) -> (361, 46.5)
  line L818 (385, 46.5) -> (365, 46.5)
  line L819 (365, 46.5) -> (365, 26.5)
  line L820 (365, 26.5) -> (385, 26.5)
  line L821 (385, 26.5) -> (385, 46.5)
  line L822 (409, 46.5) -> (389, 46.5)
  line L823 (389, 46.5) -> (389, 26.5)
  line L824 (389, 26.5) -> (409, 26.5)
  line L825 (409, 26.5) -> (409, 46.5)
  line L826 (433, 46.5) -> (413, 46.5)
  line L827 (413, 46.5) -> (413, 26.5)
  line L828 (413, 26.5) -> (433, 26.5)
  line L829 (433, 26.5) -> (433, 46.5)
  line L830 (457, 46.5) -> (437, 46.5)
  line L831 (437, 46.5) -> (437, 26.5)
  line L832 (437, 26.5) -> (457, 26.5)
  line L833 (457, 26.5) -> (457, 46.5)
  line L834 (481, 46.5) -> (461, 46.5)
  line L835 (461, 46.5) -> (461, 26.5)
  line L836 (461, 26.5) -> (481, 26.5)
  line L837 (481, 26.5) -> (481, 46.5)
  line L838 (313, 70.5) -> (293, 70.5)
  line L839 (293, 70.5) -> (293, 50.5)
  line L840 (293, 50.5) -> (313, 50.5)
  line L841 (313, 50.5) -> (313, 70.5)
  line L842 (337, 70.5) -> (317, 70.5)
  line L843 (317, 70.5) -> (317, 50.5)
  line L844 (317, 50.5) -> (337, 50.5)
  line L845 (337, 50.5) -> (337, 70.5)
  line L846 (361, 70.5) -> (341, 70.5)
  line L847 (341, 70.5) -> (341, 50.5)
  line L848 (341, 50.5) -> (361, 50.5)
  line L849 (361, 50.5) -> (361, 70.5)
  line L850 (385, 70.5) -> (365, 70.5)
  line L851 (365, 70.5) -> (365, 50.5)
  line L852 (365, 50.5) -> (385, 50.5)
  line L853 (385, 50.5) -> (385, 70.5)
  line L854 (409, 70.5) -> (389, 70.5)
  line L855 (389, 70.5) -> (389, 50.5)
  line L856 (389, 50.5) -> (409, 50.5)
  line L857 (409, 50.5) -> (409, 70.5)
  line L858 (433, 70.5) -> (413, 70.5)
  line L859 (413, 70.5) -> (413, 50.5)
  line L860 (413, 50.5) -> (433, 50.5)
  line L861 (433, 50.5) -> (433, 70.5)
  line L862 (457, 70.5) -> (437, 70.5)
  line L863 (437, 70.5) -> (437, 50.5)
  line L864 (437, 50.5) -> (457, 50.5)
  line L865 (457, 50.5) -> (457, 70.5)
  line L866 (481, 70.5) -> (461, 70.5)
  line L867 (461, 70.5) -> (461, 50.5)
  line L868 (461, 50.5) -> (481, 50.5)
  line L869 (481, 50.5) -> (481, 70.5)
  line L870 (313, 94.5) -> (293, 94.5)
  line L871 (293, 94.5) -> (293, 74.5)
  line L872 (293, 74.5) -> (313, 74.5)
  line L873 (313, 74.5) -> (313, 94.5)
  line L874 (337, 94.5) -> (317, 94.5)
  line L875 (317, 94.5) -> (317, 74.5)
  line L876 (317, 74.5) -> (337, 74.5)
  line L877 (337, 74.5) -> (337, 94.5)
  line L878 (361, 94.5) -> (341, 94.5)
  line L879 (341, 94.5) -> (341, 74.5)
  line L880 (341, 74.5) -> (361, 74.5)
  line L881 (361, 74.5) -> (361, 94.5)
  line L882 (385, 94.5) -> (365, 94.5)
  line L883 (365, 94.5) -> (365, 74.5)
  line L884 (365, 74.5) -> (385, 74.5)
  line L885 (385, 74.5) -> (385, 94.5)
  line L886 (409, 94.5) -> (389, 94.5)
  line L887 (389, 94.5) -> (389, 74.5)
  line L888 (389, 74.5) -> (409, 74.5)
  line L889 (409, 74.5) -> (409, 94.5)
  line L890 (433, 94.5) -> (413, 94.5)
  line L891 (413, 94.5) -> (413, 74.5)
  line L892 (413, 74.5) -> (433, 74.5)
  line L893 (433, 74.5) -> (433, 94.5)
  line L894 (457, 94.5) -> (437, 94.5)
  line L895 (437, 94.5) -> (437, 74.5)
  line L896 (437, 74.5) -> (457, 74.5)
  line L897 (457, 74.5) -> (457, 94.5)
  line L898 (481, 94.5) -> (461, 94.5)
  line L899 (461, 94.5) -> (461, 74.5)
  line L900 (461, 74.5) -> (481, 74.5)
  line L901 (481, 74.5) -> (481, 94.5)
  line L902 (313, 118.5) -> (293, 118.5)
  line L903 (293, 118.5) -> (293, 98.5)
  line L904 (293, 98.5) -> (313, 98.5)
  line L905 (313, 98.5) -> (313, 118.5)
  line L906 (337, 118.5) -> (317, 118.5)
  line L907 (317, 118.5) -> (317, 98.5)
  line L908 (317, 98.5) -> (337, 98.5)
  line L909 (337, 98.5) -> (337, 118.5)
  line L910 (361, 118.5) -> (341, 118.5)
  line L911 (341, 118.5) -> (341, 98.5)
  line L912 (341, 98.5) -> (361, 98.5)
  line L913 (361, 98.5) -> (361, 118.5)
  line L914 (385, 118.5) -> (365, 118.5)
  line L915 (365, 118.5) -> (365, 98.5)
  line L916 (365, 98.5) -> (385, 98.5)
  line L917 (385, 98.5) -> (385, 118.5)
  line L918 (409, 118.5) -> (389, 118.5)
  line L919 (389, 118.5) -> (389, 98.5)
  line L920 (389, 98.5) -> (409, 98.5)
  line L921 (409, 98.5) -> (409, 118.5)
  line L922 (433, 118.5) -> (413, 118.5)
  line L923 (413, 118.5) -> (413, 98.5)
  line L924 (413, 98.5) -> (433, 98.5)
  line L925 (433, 98.5) -> (433, 118.5)
  line L926 (457, 118.5) -> (437, 118.5)
  line L927 (437, 118.5) -> (437, 98.5)
  line L928 (437, 98.5) -> (457, 98.5)
  line L929 (457, 98.5) -> (457, 118.5)
  line L930 (481, 118.5) -> (461, 118.5)
  line L931 (461, 118.5) -> (461, 98.5)
  line L932 (461, 98.5) -> (481, 98.5)
  line L933 (481, 98.5) -> (481, 118.5)
  line L934 (313, 142.5) -> (293, 142.5)
  line L935 (293, 142.5) -> (293, 122.5)
  line L936 (293, 122.5) -> (313, 122.5)
  line L937 (313, 122.5) -> (313, 142.5)
  line L938 (337, 142.5) -> (317, 142.5)
  line L939 (317, 142.5) -> (317, 122.5)
  line L940 (317, 122.5) -> (337, 122.5)
  line L941 (337, 122.5) -> (337, 142.5)
  line L942 (361, 142.5) -> (341, 142.5)
  line L943 (341, 142.5) -> (341, 122.5)
  line L944 (341, 122.5) -> (361, 122.5)
  line L945 (361, 122.5) -> (361, 142.5)
  line L946 (385, 142.5) -> (365, 142.5)
  line L947 (365, 142.5) -> (365, 122.5)
  line L948 (365, 122.5) -> (385, 122.5)
  line L949 (385, 122.5) -> (385, 142.5)
  line L950 (409, 142.5) -> (389, 142.5)
  line L951 (389, 142.5) -> (389, 122.5)
  line L952 (389, 122.5) -> (409, 122.5)
  line L953 (409, 122.5) -> (409, 142.5)
  line L954 (433, 142.5) -> (413, 142.5)
  line L955 (413, 142.5) -> (413, 122.5)
  line L956 (413, 122.5) -> (433, 122.5)
  line L957 (433, 122.5) -> (433, 142.5)
  line L958 (457, 142.5) -> (437, 142.5)
  line L959 (437, 142.5) -> (437, 122.5)
  line L960 (437, 122.5) -> (457, 122.5)
  line L961 (457, 122.5) -> (457, 142.5)
  line L962 (481, 142.5) -> (461, 142.5)
  line L963 (461, 142.5) -> (461, 122.5)
  line L964 (461, 122.5) -> (481, 122.5)
  line L965 (481, 122.5) -> (481, 142.5)
  line L966 (313, 166.5) -> (293, 166.5)
  line L967 (293, 166.5) -> (293, 146.5)
  line L968 (293, 146.5) -> (313, 146.5)
  line L969 (313, 146.5) -> (313, 166.5)
  line L970 (337, 166.5) -> (317, 166.5)
  line L971 (317, 166.5) -> (317, 146.5)
  line L972 (317, 146.5) -> (337, 146.5)
  line L973 (337, 146.5) -> (337, 166.5)
  line L974 (361, 166.5) -> (341, 166.5)
  line L975 (341, 166.5) -> (341, 146.5)
  line L976 (341, 146.5) -> (361, 146.5)
  line L977 (361, 146.5) -> (361, 166.5)
  line L978 (385, 166.5) -> (365, 166.5)
  line L979 (365, 166.5) -> (365, 146.5)
  line L980 (365, 146.5) -> (385, 146.5)
  line L981 (385, 146.5) -> (385, 166.5)
  line L982 (409, 166.5) -> (389, 166.5)
  line L983 (389, 166.5) -> (389, 146.5)
  line L984 (389, 146.5) -> (409, 146.5)
  line L985 (409, 146.5) -> (409, 166.5)
  line L986 (433, 166.5) -> (413, 166.5)
  line L987 (413, 166.5) -> (413, 146.5)
  line L988 (413, 146.5) -> (433, 146.5)
  line L989 (433, 146.5) -> (433, 166.5)
  line L990 (457, 166.5) -> (437, 166.5)
  line L991 (437, 166.5) -> (437, 146.5)
  line L992 (437, 146.5) -> (457, 146.5)
  line L993 (457, 146.5) -> (457, 166.5)
  line L994 (481, 166.5) -> (461, 166.5)
  line L995 (461, 166.5) -> (461, 146.5)
  line L996 (461, 146.5) -> (481, 146.5)
  line L997 (481, 146.5) -> (481, 166.5)
  line L998 (313, 190.5) -> (293, 190.5)
  line L999 (293, 190.5) -> (293, 170.5)
  line L1000 (293, 170.5) -> (313, 170.5)
  line L1001 (313, 170.5) -> (313, 190.5)
  line L1002 (337, 190.5) -> (317, 190.5)
  line L1003 (317, 190.5) -> (317, 170.5)
  line L1004 (317, 170.5) -> (337, 170.5)
  line L1005 (337, 170.5) -> (337, 190.5)
  line L1006 (361, 190.5) -> (341, 190.5)
  line L1007 (341, 190.5) -> (341, 170.5)
  line L1008 (341, 170.5) -> (361, 170.5)
  line L1009 (361, 170.5) -> (361, 190.5)
  line L1010 (385, 190.5) -> (365, 190.5)
  line L1011 (365, 190.5) -> (365, 170.5)
  line L1012 (365, 170.5) -> (385, 170.5)
  line L1013 (385, 170.5) -> (385, 190.5)
  line L1014 (409, 190.5) -> (389, 190.5)
  line L1015 (389, 190.5) -> (389, 170.5)
  line L1016 (389, 170.5) -> (409, 170.5)
  line L1017 (409, 170.5) -> (409, 190.5)
  line L1018 (433, 190.5) -> (413, 190.5)
  line L1019 (413, 190.5) -> (413, 170.5)
  line L1020 (413, 170.5) -> (433, 170.5)
  line L1021 (433, 170.5) -> (433, 190.5)
  line L1022 (457, 190.5) -> (437, 190.5)
  line L1023 (437, 190.5) -> (437, 170.5)
  line L1024 (437, 170.5) -> (457, 170.5)
  line L1025 (457, 170.5) -> (457, 190.5)
  line L1026 (481, 190.5) -> (461, 190.5)
  line L1027 (461, 190.5) -> (461, 170.5)
  line L1028 (461, 170.5) -> (481, 170.5)
  line L1029 (481, 170.5) -> (481, 190.5)
  line L1030 (313, 214.5) -> (293, 214.5)
  line L1031 (293, 214.5) -> (293, 194.5)
  line L1032 (293, 194.5) -> (313, 194.5)
  line L1033 (313, 194.5) -> (313, 214.5)
  line L1034 (337, 214.5) -> (317, 214.5)
  line L1035 (317, 214.5) -> (317, 194.5)
  line L1036 (317, 194.5) -> (337, 194.5)
  line L1037 (337, 194.5) -> (337, 214.5)
  line L1038 (361, 214.5) -> (341, 214.5)
  line L1039 (341, 214.5) -> (341, 194.5)
  line L1040 (341, 194.5) -> (361, 194.5)
  line L1041 (361, 194.5) -> (361, 214.5)
  line L1042 (385, 214.5) -> (365, 214.5)
  line L1043 (365, 214.5) -> (365, 194.5)
  line L1044 (365, 194.5) -> (385, 194.5)
  line L1045 (385, 194.5) -> (385, 214.5)
  line L1046 (409, 214.5) -> (389, 214.5)
  line L1047 (389, 214.5) -> (389, 194.5)
  line L1048 (389, 194.5) -> (409, 194.5)
  line L1049 (409, 194.5) -> (409, 214.5)
  line L1050 (433, 214.5) -> (413, 214.5)
  line L1051 (413, 214.5) -> (413, 194.5)
  line L1052 (413, 194.5) -> (433, 194.5)
  line L1053 (433, 194.5) -> (433, 214.5)
  line L1054 (457, 214.5) -> (437, 214.5)
  line L1055 (437, 214.5) -> (437, 194.5)
  line L1056 (437, 194.5) -> (457, 194.5)
  line L1057 (457, 194.5) -> (457, 214.5)
  line L1058 (481, 214.5) -> (461, 214.5)
  line L1059 (461, 214.5) -> (461, 194.5)
  line L1060 (461, 194.5) -> (481, 194.5)
  line L1061 (481, 194.5) -> (481, 214.5)
  line L1062 (313, 238.5) -> (293, 238.5)
  line L1063 (293, 238.5) -> (293, 218.5)
  line L1064 (293, 218.5) -> (313, 218.5)
  line L1065 (313, 218.5) -> (313, 238.5)
  line L1066 (337, 238.5) -> (317, 238.5)
  line L1067 (317, 238.5) -> (317, 218.5)
  line L1068 (317, 218.5) -> (337, 218.5)
  line L1069 (337, 218.5) -> (337, 238.5)
  line L1070 (361, 238.5) -> (341, 238.5)
  line L1071 (341, 238.5) -> (341, 218.5)
  line L1072 (341, 218.5) -> (361, 218.5)
  line L1073 (361, 218.5) -> (361, 238.5)
  line L1074 (385, 238.5) -> (365, 238.5)
  line L1075 (365, 238.5) -> (365, 218.5)
  line L1076 (365, 218.5) -> (385, 218.5)
  line L1077 (385, 218.5) -> (385, 238.5)
  line L1078 (409, 238.5) -> (389, 238.5)
  line L1079 (389, 238.5) -> (389, 218.5)
  line L1080 (389, 218.5) -> (409, 218.5)
  line L1081 (409, 218.5) -> (409, 238.5)
  line L1082 (433, 238.5) -> (413, 238.5)
  line L1083 (413, 238.5) -> (413, 218.5)
  line L1084 (413, 218.5) -> (433, 218.5)
  line L1085 (433, 218.5) -> (433, 238.5)
  line L1086 (457, 238.5) -> (437, 238.5)
  line L1087 (437, 238.5) -> (437, 218.5)
  line L1088 (437, 218.5) -> (457, 218.5)
  line L1089 (457, 218.5) -> (457, 238.5)
  line L1090 (481, 238.5) -> (461, 238.5)
  line L1091 (461, 238.5) -> (461, 218.5)
  line L1092 (461, 218.5) -> (481, 218.5)
  line L1093 (481, 218.5) -> (481, 238.5)
  line L1094 (313, 262.5) -> (293, 262.5)
  line L1095 (293, 262.5) -> (293, 242.5)
  line L1096 (293, 242.5) -> (313, 242.5)
  line L1097 (313, 242.5) -> (313, 262.5)
  line L1098 (337, 262.5) -> (317, 262.5)
  line L1099 (317, 262.5) -> (317, 242.5)
  line L1100 (317, 242.5) -> (337, 242.5)
  line L1101 (337, 242.5) -> (337, 262.5)
  line L1102 (361, 262.5) -> (341, 262.5)
  line L1103 (341, 262.5) -> (341, 242.5)
  line L1104 (341, 242.5) -> (361, 242.5)
  line L1105 (361, 242.5) -> (361, 262.5)
  line L1106 (385, 262.5) -> (365, 262.5)
  line L1107 (365, 262.5) -> (365, 242.5)
  line L1108 (365, 242.5) -> (385, 242.5)
  line L1109 (385, 242.5) -> (385, 262.5)
  line L1110 (409, 262.5) -> (389, 262.5)
  line L1111 (389, 262.5) -> (389, 242.5)
  line L1112 (389, 242.5) -> (409, 242.5)
  line L1113 (409, 242.5) -> (409, 262.5)
  line L1114 (433, 262.5) -> (413, 262.5)
  line L1115 (413, 262.5) -> (413, 242.5)
  line L1116 (413, 242.5) -> (433, 242.5)
  line L1117 (433, 242.5) -> (433, 262.5)
  line L1118 (457, 262.5) -> (437, 262.5)
  line L1119 (437, 262.5) -> (437, 242.5)
  line L1120 (437, 242.5) -> (457, 242.5)
  line L1121 (457, 242.5) -> (457, 262.5)
  line L1122 (481, 262.5) -> (461, 262.5)
  line L1123 (461, 262.5) -> (461, 242.5)
  line L1124 (461, 242.5) -> (481, 242.5)
  line L1125 (481, 242.5) -> (481, 262.5)
  line L1126 (313, 286.5) -> (293, 286.5)
  line L1127 (293, 286.5) -> (293, 266.5)
  line L1128 (293, 266.5) -> (313, 266.5)
  line L1129 (313, 266.5) -> (313, 286.5)
  line L1130 (337, 286.5) -> (317, 286.5)
  line L1131 (317, 286.5) -> (317, 266.5)
  line L1132 (317, 266.5) -> (337, 266.5)
  line L1133 (337, 266.5) -> (337, 286.5)
  line L1134 (361, 286.5) -> (341, 286.5)
  line L1135 (341, 286.5) -> (341, 266.5)
  line L1136 (341, 266.5) -> (361, 266.5)
  line L1137 (361, 266.5) -> (361, 286.5)
  line L1138 (385, 286.5) -> (365, 286.5)
  line L1139 (365, 286.5) -> (365, 266.5)
  line L1140 (365, 266.5) -> (385, 266.5)
  line L1141 (385, 266.5) -> (385, 286.5)
  line L1142 (409, 286.5) -> (389, 286.5)
  line L1143 (389, 286.5) -> (389, 266.5)
  line L1144 (389, 266.5) -> (409, 266.5)
  line L1145 (409, 266.5) -> (409, 286.5)
  line L1146 (433, 286.5) -> (413, 286.5)
  line L1147 (413, 286.5) -> (413, 266.5)
  line L1148 (413, 266.5) -> (433, 266.5)
  line L1149 (433, 266.5) -> (433, 286.5)
  line L1150 (457, 286.5) -> (437, 286.5)
  line L1151 (437, 286.5) -> (437, 266.5)
  line L1152 (437, 266.5) -> (457, 266.5)
  line L1153 (457, 266.5) -> (457, 286.5)
  line L1154 (481, 286.5) -> (461, 286.5)
  line L1155 (461, 286.5) -> (461, 266.5)
  line L1156 (461, 266.5) -> (481, 266.5)
  line L1157 (481, 266.5) -> (481, 286.5)
  line L1158 (313, 310.5) -> (293, 310.5)
  line L1159 (293, 310.5) -> (293, 290.5)
  line L1160 (293, 290.5) -> (313, 290.5)
  line L1161 (313, 290.5) -> (313, 310.5)
  line L1162 (337, 310.5) -> (317, 310.5)
  line L1163 (317, 310.5) -> (317, 290.5)
  line L1164 (317, 290.5) -> (337, 290.5)
  line L1165 (337, 290.5) -> (337, 310.5)
  line L1166 (361, 310.5) -> (341, 310.5)
  line L1167 (341, 310.5) -> (341, 290.5)
  line L1168 (341, 290.5) -> (361, 290.5)
  line L1169 (361, 290.5) -> (361, 310.5)
  line L1170 (385, 310.5) -> (365, 310.5)
  line L1171 (365, 310.5) -> (365, 290.5)
  line L1172 (365, 290.5) -> (385, 290.5)
  line L1173 (385, 290.5) -> (385, 310.5)
  line L1174 (409, 310.5) -> (389, 310.5)
  line L1175 (389, 310.5) -> (389, 290.5)
  line L1176 (389, 290.5) -> (409, 290.5)
  line L1177 (409, 290.5) -> (409, 310.5)
  line L1178 (433, 310.5) -> (413, 310.5)
  line L1179 (413, 310.5) -> (413, 290.5)
  line L1180 (413, 290.5) -> (433, 290.5)
  line L1181 (433, 290.5) -> (433, 310.5)
  line L1182 (457, 310.5) -> (437, 310.5)
  line L1183 (437, 310.5) -> (437, 290.5)
  line L1184 (437, 290.5) -> (457, 290.5)
  line L1185 (457, 290.5) -> (457, 310.5)
  line L1186 (481, 310.5) -> (461, 310.5)
  line L1187 (461, 310.5) -> (461, 290.5)
  line L1188 (461, 290.5) -> (481, 290.5)
  line L1189 (481, 290.5) -> (481, 310.5)
  line L1190 (313, 334.5) -> (293, 334.5)
  line L1191 (293, 334.5) -> (293, 314.5)
  line L1192 (293, 314.5) -> (313, 314.5)
  line L1193 (313, 314.5) -> (313, 334.5)
  line L1194 (337, 334.5) -> (317, 334.5)
  line L1195 (317, 334.5) -> (317, 314.5)
  line L1196 (317, 314.5) -> (337, 314.5)
  line L1197 (337, 314.5) -> (337, 334.5)
  line L1198 (361, 334.5) -> (341, 334.5)
  line L1199 (341, 334.5) -> (341, 314.5)
  line L1200 (341, 314.5) -> (361, 314.5)
  line L1201 (361, 314.5) -> (361, 334.5)
  line L1202 (385, 334.5) -> (365, 334.5)
  line L1203 (365, 334.5) -> (365, 314.5)
  line L1204 (365, 314.5) -> (385, 314.5)
  line L1205 (385, 314.5) -> (385, 334.5)
  line L1206 (409, 334.5) -> (389, 334.5)
  line L1207 (389, 334.5) -> (389, 314.5)
  line L1208 (389, 314.5) -> (409, 314.5)
  line L1209 (409, 314.5) -> (409, 334.5)
  line L1210 (433, 334.5) -> (413, 334.5)
  line L1211 (413, 334.5) -> (413, 314.5)
  line L1212 (413, 314.5) -> (433, 314.5)
  line L1213 (433, 314.5) -> (433, 334.5)
  line L1214 (457, 334.5) -> (437, 334.5)
  line L1215 (437, 334.5) -> (437, 314.5)
  line L1216 (437, 314.5) -> (457, 314.5)
  line L1217 (457, 314.5) -> (457, 334.5)
  line L1218 (481, 334.5) -> (461, 334.5)
  line L1219 (461, 334.5) -> (461, 314.5)
  line L1220 (461, 314.5) -> (481, 314.5)
  line L1221 (481, 314.5) -> (481, 334.5)
  line L1222 (313, 358.5) -> (293, 358.5)
  line L1223 (293, 358.5) -> (293, 338.5)
  line L1224 (293, 338.5) -> (313, 338.5)
  line L1225 (313, 338.5) -> (313, 358.5)
  line L1226 (337, 358.5) -> (317, 358.5)
  line L1227 (317, 358.5) -> (317, 338.5)
  line L1228 (317, 338.5) -> (337, 338.5)
  line L1229 (337, 338.5) -> (337, 358.5)
  line L1230 (361, 358.5) -> (341, 358.5)
  line L1231 (341, 358.5) -> (341, 338.5)
  line L1232 (341, 338.5) -> (361, 338.5)
  line L1233 (361, 338.5) -> (361, 358.5)
  line L1234 (385, 358.5) -> (365, 358.5)
  line L1235 (365, 358.5) -> (365, 338.5)
  line L1236 (365, 338.5) -> (385, 338.5)
  line L1237 (385, 338.5) -> (385, 358.5)
  line L1238 (409, 358.5) -> (389, 358.5)